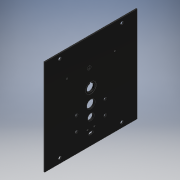
# Autodesk Inventor part: Structure_+X
Saved by Autodesk Inventor 2018 (Build 220112000, 112)
## iProperties
Created: 2018-07-04
Part Number: Structure_+X
Material: Aluminum 6061
Document SubType Name: Modeling
Designer: Bradley
Density: 2.7 g/cm^3
Appearance: Anodized - Dark Gray
Mass: 30.0277 g
Surface Area: 203.66 cm^2
Volume: 11.1214 cm^3
Author: Bradley
Autodesk Inventor part; units mm, degrees
ref_plane "YZ Plane" through (0, 0, 0) normal (1, 0, 0) x (0, 1, 0)
ref_plane "XZ Plane" through (0, 0, 0) normal (0, 1, 0) x (-1, 0, 0)
ref_plane "XY Plane" through (0, 0, 0) normal (0, 0, 1) x (1, 0, 0)
sketch "Sketch1" plane through (0, 0, 0) normal (1, 0, 0) x (0, 1, 0)
  line L0 (-48.5, -50) -> (48.5, -50)
  line L1 (48.5, -50) -> (48.5, 50)
  line L2 (48.5, 50) -> (-48.5, 50)
  line L3 (-48.5, 50) -> (-48.5, -50)
  line L4 (-48.5, -50) -> (48.5, 50) construction
  line L5 (48.5, -50) -> (-48.5, 50) construction
  point P0 (0, 0)
  dimension "d0" = 97
  dimension "d1" = 100
  constraints: 12 end point, 2 midpoint, 2 parallel, 1 horizontal, 1 perpendicular
  measures "d0" distance of L2.end L1.end
  measures "d1" distance of L1.end L0.end
extrude "Extrusion1" add sketch "Sketch1" along normal mid plane 1
sketch "Sketch2" plane through (0.5, 0, 0) normal (1, 0, 0) x (0, 0, -1)
  line L0 (45, -32.5) -> (-45, -32.5) construction
  line L1 (-45, -32.5) -> (-45, 32.5) construction
  line L2 (-45, 32.5) -> (45, 32.5) construction
  line L3 (45, 32.5) -> (45, -32.5) construction
  line L4 (45, -32.5) -> (-45, 32.5) construction
  line L5 (-45, -32.5) -> (45, 32.5) construction
  point P0 (0, 0)
  dimension "d5" = 90
  dimension "d6" = 65
  constraints: 12 end point, 4 coincident, 2 midpoint, 2 parallel, 1 horizontal, 1 perpendicular
  measures "d5" distance of L1.end L2.end
  measures "d6" distance of L0.end L1.end
hole "Hole1" at (0.5, -32.5, 45) at (0.5, 32.5, 45) at (0.5, 32.5, -45) at (0.5, -32.5, -45) direction (-1, 0, 0) diameter 3.2 end through all clearance for "Socket Head Cap Screw" size "M3" standard "Ansi Metric M Profile"
sketch "Sketch3" plane through (0.5, 0, 0) normal (1, 0, 0) x (0, 0, -1)
  circle A0 centre (-2.5, 0) radius 4.05
  line L0 (-6.4651, -0.825) -> (-7.3, -0.825)
  line L1 (-7.7, -0.425) -> (-7.7, 0.425)
  line L2 (-7.3, 0.825) -> (-6.4651, 0.825)
  line L3 (-6.4651, 0.825) -> (-6.4651, -0.825)
  circle A1 centre (12.35, 0) radius 4
  line L4 (-7.5, -0.75) -> (-6.4651, -0.75) construction
  line L5 (-6.4651, -0.75) -> (-6.4651, 0.75) construction
  line L6 (-6.4651, 0.75) -> (-7.5, 0.75) construction
  line L7 (-7.5, 0.75) -> (-7.5, -0.75) construction
  arc A2 (-7.7, -0.425) -> (-7.3, -0.825) centre (-7.3, -0.425) ccw
  arc A3 (-7.3, 0.825) -> (-7.7, 0.425) centre (-7.3, 0.425) ccw
  circle A4 centre (-2.5, 0) radius 5.5 construction
  circle A5 centre (24, 0) radius 3
  circle A6 centre (-21.5, -1.75) radius 1.5
  line L8 (38.6, -1) -> (38.6, 1) construction
  line L9 (39.6, -1) -> (39.6, 1)
  line L10 (37.6, 1) -> (37.6, -1)
  arc A7 (37.6, -1) -> (39.6, -1) centre (38.6, -1) ccw
  arc A8 (39.6, 1) -> (37.6, 1) centre (38.6, 1) ccw
  line L11 (15, -15) -> (30, -15) construction
  line L12 (30, -15) -> (30, 15) construction
  line L13 (30, 15) -> (15, 15) construction
  line L14 (15, 15) -> (15, -15) construction
  circle A9 centre (15, -15) radius 1
  circle A10 centre (15, 15) radius 1
  circle A11 centre (30, 15) radius 1
  circle A12 centre (30, -15) radius 1
  point P0 (0, 0)
  point P1 (-7.7, 0.825)
  point P2 (-7.7, -0.825)
  point P3 (-7.5, 0)
  point P4 (38.6, 0)
  point P5 (15, 0)
  dimension "d14" = 2.5
  dimension "d15" = 8.1
  dimension "d16" = 1.65
  dimension "d17" = 5.2
  dimension "d18" = 12.35
  dimension "d19" = 8
  dimension "d26" = 5
  dimension "d27" = 1.5
  dimension "d28" = 0.4
  dimension "d29" = 11
  dimension "d43" = 6
  dimension "d44" = 26.5
  dimension "d48" = 1.75
  dimension "d49" = 21.5
  dimension "d50" = 3
  dimension "d51" = 38.6
  dimension "d52" = 2
  dimension "d53" = 2
  dimension "d83" = 15
  dimension "d84" = 30
  dimension "d85" = 15
  dimension "d86" = 2
  constraints: 32 end point, 13 centre point, 10 point on circle, 8 tangent, 7 parallel, 6 horizontal alignment, 5 coincident, 4 equal radius, 4 point on line, 3 horizontal, 3 midpoint, 3 perpendicular, 1 collinear, 1 vertical
  measures "d14" distance of point (0, 0) A0.centre
  measures "d15" diameter of A0
  measures "d16" distance of point (-7.7, -0.825) point (-7.7, 0.825)
  measures "d17" distance from line of A0.centre L1
  measures "d18" distance of A1.centre point (0, 0)
  measures "d19" diameter of A1
  measures "d26" distance from line of A0.centre L7
  measures "d27" distance of L6.end L4.start
  measures "d28" radius of A2
  measures "d29" diameter of A4
  measures "d43" diameter of A5
  measures "d44" distance of A5.centre A4.centre
  measures "d48" vertical distance of A4.centre A6.centre
  measures "d49" horizontal distance of point (0, 0) A6.centre
  measures "d50" diameter of A6
  measures "d51" distance from line of point (0, 0) L8
  measures "d52" distance of L8.start L8.end
  measures "d53" distance between parallel lines of L9 L10
  measures "d83" distance of L13.end L12.end
  measures "d84" distance of L12.end L11.end
  measures "d85" distance from line of L14 point (0, 0)
  measures "d86" diameter of A9
extrude "Extrusion2" cut sketch "Sketch3" against normal through all
sketch "Sketch4" plane through (0.5, 0, 0) normal (1, 0, 0) x (0, 0, -1)
  circle A0 centre (12.35, 0) radius 4 projected
  arc A1 (-6.4651, -0.825) -> (-6.4651, 0.825) centre (-2.5, 0) ccw projected
  line L0 (-6.4651, -0.825) -> (-7.3, -0.825) projected
  line L1 (-7.7, -0.425) -> (-7.7, 0.425) projected
  line L2 (-7.3, 0.825) -> (-6.4651, 0.825) projected
  circle A2 centre (45, 32.5) radius 1.6 projected
  circle A3 centre (-45, -32.5) radius 1.6 projected
  circle A4 centre (-45, 32.5) radius 1.6 projected
  circle A5 centre (45, -32.5) radius 1.6 projected
  line L3 (50, -48.5) -> (50, 48.5) projected
  line L4 (50, 48.5) -> (-50, 48.5) projected
  line L5 (-50, 48.5) -> (-50, -48.5) projected
  line L6 (-50, -48.5) -> (50, -48.5) projected
  circle A6 centre (-2.5, 0) radius 5.6
  arc A7 (-7.7, -0.425) -> (-7.3, -0.825) centre (-7.3, -0.425) ccw projected
  arc A8 (-7.3, 0.825) -> (-7.7, 0.425) centre (-7.3, 0.425) ccw projected
  point P0 (0, 0)
  dimension "d22" = 11.2
  constraints: 1 centre point, 1 coincident
  measures "d22" diameter of A6
extrude "Extrusion3" cut sketch "Sketch4" against normal blind 0.3 contours A6
sketch "Sketch8" plane through (0.5, 0, 0) normal (1, 0, 0) x (0, 0, -1)
  line L0 (34.1, -3.5714) -> (34.1, 3.5714) construction
  arc A0 (39.6, 1) -> (37.6, 1) centre (38.6, 1) ccw projected
  circle A1 centre (0, 0) radius 39 construction
  line L1 (38.6, 5.5714) -> (38.6, 5.5714) construction
  point P0 (34.1, 0)
  dimension "d55" = 4.5
  dimension "d87" = 78
  dimension "d88" = 2
  constraints: 4 end point, 3 coincident, 2 point on circle, 2 vertical, 1 centre point, 1 horizontal alignment, 1 midpoint, 1 point on line
  measures "d55" distance from line of L0 A0.centre
  measures "d87" diameter of A1
  measures "d88" vertical distance of L1.end L0.end
hole "Hole2" at (0.5, -3.5714, -34.1) at (0.5, 3.5714, -34.1) direction (-1, 0, 0) diameter 1.567 end through all thread size "M2x0.4" class "6H" standard "ANSI Metric M Profile"
sketch "Sketch5" plane through (-0.5, 0, 0) normal (-1, 0, 0) x (0, 0, 1)
  circle A0 centre (-12.35, 0) radius 4 projected
  arc A1 (6.4651, 0.825) -> (6.4651, -0.825) centre (2.5, 0) ccw projected
  line L0 (6.4651, 0.825) -> (7.3, 0.825) projected
  arc A2 (7.7, 0.425) -> (7.3, 0.825) centre (7.3, 0.425) ccw projected
  line L1 (7.7, 0.425) -> (7.7, -0.425) projected
  arc A3 (7.3, -0.825) -> (7.7, -0.425) centre (7.3, -0.425) ccw projected
  line L2 (7.3, -0.825) -> (6.4651, -0.825) projected
  circle A4 centre (-45, 32.5) radius 1.6 projected
  circle A5 centre (45, -32.5) radius 1.6 projected
  circle A6 centre (45, 32.5) radius 1.6 projected
  circle A7 centre (-45, -32.5) radius 1.6 projected
  line L3 (-50, 48.5) -> (-50, -48.5) projected
  line L4 (-50, -48.5) -> (50, -48.5) projected
  line L5 (50, -48.5) -> (50, 48.5) projected
  line L6 (50, 48.5) -> (-50, 48.5) projected
  line L7 (40, 45.9) -> (-40, 45.9)
  line L8 (-40, 45.9) -> (-40, 41.9)
  line L9 (-40, 41.9) -> (40, 41.9)
  line L10 (40, 41.9) -> (40, 45.9)
  line L11 (-40, -45.9) -> (40, -45.9)
  line L12 (40, -45.9) -> (40, -41.9)
  line L13 (40, -41.9) -> (-40, -41.9)
  line L14 (-40, -41.9) -> (-40, -45.9)
  line L15 (50, -48.5) -> (50, 48.5) construction
  line L16 (50, 0) -> (-50, 0) construction
  line L17 (-50, -48.5) -> (-50, 48.5) construction
  circle A8 centre (2.5, 0) radius 7.5
  line L18 (40, 41.9) -> (8.6628, 4.2743)
  line L19 (8.6628, -4.2743) -> (40, -41.9)
  line L20 (-40, -41.9) -> (-3.9256, -3.8681)
  line L21 (-40, 41.9) -> (-3.9256, 3.8681)
  line L22 (-1.0235, 6.6208) -> (-34.4868, 41.9)
  line L23 (-34.4868, -41.9) -> (-1.0235, -6.6208)
  line L24 (34.7944, 41.9) -> (5.5892, 6.8342)
  circle A9 centre (2.5, 0) radius 5.6 projected
  line L25 (2.5, 0) -> (37.3972, 41.9) construction
  line L26 (2.5, 0) -> (-37.2434, 41.9) construction
  line L27 (34.7944, -41.9) -> (5.5892, -6.8342)
  circle A10 centre (-24, 0) radius 3 projected
  circle A11 centre (-12.35, 0) radius 5
  circle A12 centre (-24, 0) radius 4
  circle A13 centre (-34.1, -3.5714) radius 0.7835 projected
  circle A14 centre (-34.1, 3.5714) radius 0.7835 projected
  circle A15 centre (-12.35, 0) radius 4 projected
  arc A16 (-37.6, 1) -> (-39.6, 1) centre (-38.6, 1) ccw projected
  line L28 (-37.6, 1) -> (-37.6, -1) projected
  arc A17 (-39.6, -1) -> (-37.6, -1) centre (-38.6, -1) ccw projected
  line L29 (-39.6, -1) -> (-39.6, 1) projected
  arc A18 (6.4651, 0.825) -> (6.4651, -0.825) centre (2.5, 0) ccw projected
  line L30 (6.4651, 0.825) -> (7.3, 0.825) projected
  arc A19 (7.7, 0.425) -> (7.3, 0.825) centre (7.3, 0.425) ccw projected
  line L31 (7.7, 0.425) -> (7.7, -0.425) projected
  arc A20 (7.3, -0.825) -> (7.7, -0.425) centre (7.3, -0.425) ccw projected
  line L32 (7.3, -0.825) -> (6.4651, -0.825) projected
  circle A21 centre (21.5, -1.75) radius 1.5 projected
  circle A22 centre (-24, 0) radius 3 projected
  circle A23 centre (-45, 32.5) radius 1.6 projected
  circle A24 centre (45, -32.5) radius 1.6 projected
  circle A25 centre (45, 32.5) radius 1.6 projected
  circle A26 centre (-45, -32.5) radius 1.6 projected
  line L33 (-50, 48.5) -> (-50, -48.5) projected
  line L34 (-50, -48.5) -> (50, -48.5) projected
  line L35 (50, -48.5) -> (50, 48.5) projected
  line L36 (50, 48.5) -> (-50, 48.5) projected
  line L37 (-32.1, 3.5714) -> (-32.1, -3.5714)
  arc A27 (-36.1, -3.5714) -> (-32.1, -3.5714) centre (-34.1, -3.5714) ccw
  line L38 (-36.1, -3.5714) -> (-36.1, 3.5714)
  arc A28 (-32.1, 3.5714) -> (-36.1, 3.5714) centre (-34.1, 3.5714) ccw
  circle A29 centre (-34.1, 3.5714) radius 0.7835 projected
  circle A30 centre (21.5, -1.75) radius 1.5 projected
  circle A31 centre (21.5, -1.75) radius 3
  point P0 (0, 0)
  point P1 (0, 41.9)
  point P2 (0, 0)
  dimension "d36" = 15
  dimension "d33" = 45.9
  dimension "d34" = 4
  dimension "d35" = 80
  dimension "d37" = 4
  dimension "d38" = 4
  dimension "d45" = 10
  dimension "d46" = 8
  dimension "d47" = 2.35
  dimension "d67" = 2
  dimension "d70" = 6
  constraints: 42 end point, 9 parallel, 6 point on line, 5 centre point, 4 coincident, 4 equal length, 4 midpoint, 4 point on circle, 4 tangent, 2 concentric, 2 horizontal, 2 perpendicular, 1 vertical, 1 vertical alignment, 16 other
  measures "d33" distance between parallel lines of L16 L7
  measures "d34" distance of L9.end L7.start
  measures "d35" distance of L7.start L7.end
  measures "d37" distance between parallel lines of L24 L18
  measures "d38" distance between parallel lines of L21 L22
  measures "d45" diameter of A11
  measures "d46" diameter of A12
  measures "d67" radius of A28
  measures "d70" diameter of A31
extrude "Extrusion4" add sketch "Sketch5" along normal blind 1 contours L10 L9 L8 L7 | L18 A8 L24 L9 | L9 L22 A8 L21 | A8 | A8 L23 L13 L20 | L19 L13 L27 A8 | L13 L12 L11 L14 | A9 | A11 | A12 | A21 | L37 A27 L38 A28 | A31
chamfer "Chamfer1" distance 0.5 angle 45 13 edges at (0.5, 0, -8.35) (-1.5, 0, -16.35) (-1.5, 0, -27) (0.5, 0, -21) (0.5, 0, -37.6) (0.5, 2, -38.6) (0.5, 0, -39.6) (0.5, -2, -38.6) (0.5, -1.75, 23) (0.5, 15, -14) (0.5, 15, -29) (0.5, -15, -29) (0.5, -15, -14)
fillet "Fillet3" radius 2 16 edges at (-1, 41.9, 40) (-1, 41.9, 34.7944) (-1, 41.9, -40) (-1, 41.9, -34.4868) (-1, 6.8342, 5.5892) (-1, 6.6208, -1.0235) (-1, 4.2743, 8.6628) (-1, -4.2743, 8.6628) (-1, -41.9, 40) (-1, -41.9, 34.7944) (-1, -6.8342, 5.5892) (-1, -6.6208, -1.0235) (-1, 3.8681, -3.9256) (-1, -3.8681, -3.9256) (-1, -41.9, -40) (-1, -41.9, -34.4868)
fillet "Fillet3" radius 1 4 edges at (-1, -45.9, -40) (-1, -45.9, 40) (-1, 45.9, -40) (-1, 45.9, 40)
sketch "Sketch10" plane through (0.5, 0, 0) normal (1, 0, 0) x (0, 0, -1)
  line L0 (-2.5, 0) -> (-37.3972, 41.9) projected
  circle A0 centre (34.1, -3.5714) radius 0.7835 projected
  line L1 (-23.3841, 25.0749) -> (-23.3841, -25.0749) construction
  circle A1 centre (0, 0) radius 34.2865 construction
  constraints: 3 coincident, 3 point on circle, 2 end point, 1 centre point, 1 point on line, 1 vertical
hole "Hole3" at (0.5, -25.0749, 23.3841) at (0.5, 25.0749, 23.3841) direction (-1, 0, 0) diameter 1.567 end through all thread size "M2x0.4" class "6H" standard "ANSI Metric M Profile"
equation "\"d37\" = d34"
equation "\"d38\" = d34"
body "Solid1"
